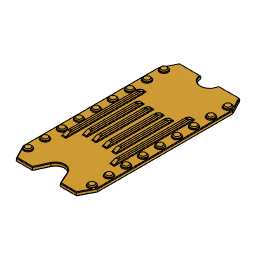
Spojka v7 (Autodesk Fusion 360 design; units mm, degrees)
Autodesk Fusion 360 part; units mm, degrees
note: some values were not read from the file. Set by a fixed rule: which sketch regions a step uses.
sketch "Sketch1" plane through (0, 0, 0) normal (0, 0, 1) x (1, 0, 0)
  line L0 (13.175, -28.845) -> (-13.175, -28.845)
  line L1 (-13.175, -28.845) -> (-13.175, 28.845)
  line L2 (-13.175, 28.845) -> (13.175, 28.845)
  line L3 (13.175, 28.845) -> (13.175, -28.845)
  line L4 (13.175, -28.845) -> (-13.175, 28.845) construction
  line L5 (-13.175, -28.845) -> (13.175, 28.845) construction
  circle A0 centre (0, 28.845) radius 3.15
  circle A1 centre (0, -25.665) radius 3.15
  line L6 (-2.869, -24.3645) -> (-4.9, -28.845)
  line L7 (2.869, -24.3645) -> (4.9, -28.845)
  line L8 (-13.175, 23.845) -> (-10.595, 28.845)
  line L9 (0, 2.5) -> (0, 20)
  line L10 (13.175, 23.845) -> (10.595, 28.845)
  line L11 (20, 0) -> (2.5, 0)
  line L12 (-13.175, -23.845) -> (-10.595, -28.845)
  line L13 (13.175, -23.845) -> (10.595, -28.845)
  circle A2 centre (-11.295, 0) radius 1.25
  circle A3 centre (-11.295, -24) radius 1.25
  circle A4 centre (-11.295, -18) radius 1.25
  circle A5 centre (-11.295, -12) radius 1.25
  circle A6 centre (-11.295, -6) radius 1.25
  circle A7 centre (-11.295, 6) radius 1.25
  circle A8 centre (-11.295, 12) radius 1.25
  circle A9 centre (-11.295, 18) radius 1.25
  circle A10 centre (-11.295, 24) radius 1.25
  circle A11 centre (11.295, 24) radius 1.25
  circle A12 centre (11.295, 18) radius 1.25
  circle A13 centre (11.295, 12) radius 1.25
  circle A14 centre (11.295, 6) radius 1.25
  circle A15 centre (11.295, 0) radius 1.25
  circle A16 centre (11.295, -6) radius 1.25
  circle A17 centre (11.295, -12) radius 1.25
  circle A18 centre (11.295, -18) radius 1.25
  circle A19 centre (11.295, -24) radius 1.25
  line L14 (-7.925, -14) -> (-9.175, -14)
  line L15 (-9.175, -14) -> (-9.175, 14)
  line L16 (-9.175, 14) -> (-7.925, 14)
  line L17 (-7.925, 14) -> (-7.925, -14)
  line L18 (-7.925, -14) -> (-9.175, 14) construction
  line L19 (-9.175, -14) -> (-7.925, 14) construction
  line L20 (-4.575, -10) -> (-5.825, -10)
  line L21 (-5.825, -10) -> (-5.825, 10)
  line L22 (-5.825, 10) -> (-4.575, 10)
  line L23 (-4.575, 10) -> (-4.575, -10)
  line L24 (-4.575, -10) -> (-5.825, 10) construction
  line L25 (-5.825, -10) -> (-4.575, 10) construction
  line L26 (-1.225, -10) -> (-2.475, -10)
  line L27 (-2.475, -10) -> (-2.475, 10)
  line L28 (-2.475, 10) -> (-1.225, 10)
  line L29 (-1.225, 10) -> (-1.225, -10)
  line L30 (-1.225, -10) -> (-2.475, 10) construction
  line L31 (-2.475, -10) -> (-1.225, 10) construction
  line L32 (9.175, -14) -> (9.175, 14)
  line L33 (9.175, 14) -> (7.925, 14)
  line L34 (7.925, -14) -> (9.175, -14)
  line L35 (7.925, 14) -> (7.925, -14)
  line L36 (4.575, 10) -> (4.575, -10)
  line L37 (4.575, -10) -> (5.825, -10)
  line L38 (5.825, 10) -> (4.575, 10)
  line L39 (5.825, -10) -> (5.825, 10)
  line L40 (1.225, 10) -> (1.225, -10)
  line L41 (1.225, -10) -> (2.475, -10)
  line L42 (2.475, 10) -> (1.225, 10)
  line L43 (2.475, -10) -> (2.475, 10)
  point P0 (-8.55, 0)
  point P1 (-5.2, 0)
  point P2 (-1.85, 0)
  dimension "d1" = 26.35
  dimension "d2" = 57.69
  dimension "d3" = 6.3
  dimension "d4" = 9.8
  dimension "d5" = 6.33
  dimension "d6" = 2.58
  dimension "d7" = 5
  dimension "d8" = 2.5
  dimension "d9" = 1.88
  dimension "d12" = 0
  dimension "d13" = 6
  dimension "d14" = 1.25
  dimension "d15" = 28
  dimension "d16" = 1.25
  dimension "d17" = 20
  dimension "d18" = 4
  dimension "d19" = 2.1
  dimension "d20" = 2.1
  constraint horizontal L0
  constraint perpendicular L0 L1
  constraint parallel L0 L2
  constraint parallel L1 L3
  constraint coincident L4 origin
  constraint coincident L5 origin
  constraint midpoint L2 A0.centre
  constraint equal A0 A1
  constraint coincident A1 L6.start
  constraint coincident L0 L6.end
  constraint coincident A1 L7.start
  constraint coincident L0 L7.end
  constraint tangent A1 L7
  constraint tangent A1 L6
  constraint equal L6 L7
  constraint vertical origin A1.centre
  constraint coincident L1 L8.start
  constraint coincident L2 L8.end
  constraint symmetric L8.start L9 L10.start
  constraint symmetric L8.end L9 L10.end
  constraint symmetric L8.start L11 L12.start
  constraint symmetric L8.end L11 L12.end
  constraint symmetric L10.start L11 L13.start
  constraint symmetric L10.end L11 L13.end
  constraint horizontal origin A2.centre
  constraint symmetric L9 A2 A15
  constraint symmetric L9 A3 A19
  constraint symmetric L9 A4 A18
  constraint symmetric L9 A5 A17
  constraint symmetric L9 A6 A16
  constraint symmetric L9 A7 A14
  constraint symmetric L9 A8 A13
  constraint symmetric L9 A9 A12
  constraint symmetric L9 A10 A11
  constraint horizontal L14
  constraint perpendicular L14 L15
  constraint parallel L14 L16
  constraint parallel L15 L17
  constraint coincident L18 P0
  constraint coincident L19 P0
  constraint horizontal L20
  constraint perpendicular L20 L21
  constraint parallel L20 L22
  constraint parallel L21 L23
  constraint coincident L24 P1
  constraint coincident L25 P1
  constraint horizontal origin P1
  constraint horizontal origin P0
  constraint horizontal L26
  constraint perpendicular L26 L27
  constraint parallel L26 L28
  constraint parallel L27 L29
  constraint coincident L30 P2
  constraint coincident L31 P2
  constraint horizontal origin P2
  constraint equal L22 L28
  constraint equal L23 L27
  constraint symmetric L9 L14.start L34.start
  constraint symmetric L9 L14.end L32.start
  constraint symmetric L9 L15.end L32.end
  constraint symmetric L9 L16.end L33.end
  constraint symmetric L9 L20.start L36.end
  constraint symmetric L9 L20.end L37.end
  constraint symmetric L9 L21.end L38.start
  constraint symmetric L9 L22.end L36.start
  constraint symmetric L9 L26.start L40.end
  constraint symmetric L9 L26.end L41.end
  constraint symmetric L9 L27.end L42.start
  constraint symmetric L9 L28.end L40.start
  measures "d1" distance of L1.end L2.end
  measures "d2" distance of L0.end L1.end
  measures "d3" diameter of A0
  measures "d4" distance of L6.end L7.end
  measures "d6" distance of L1.end L8.end
  measures "d7" distance of L1.end L8.start
  measures "d8" diameter of A2
  measures "d9" distance of L1 A2.centre
  measures "d14" distance of L15.end L16.end
  measures "d15" distance of L14.end L15.end
  measures "d16" distance of L21.end L22.end
  measures "d17" distance of L20.end L21.end
  measures "d18" distance of L1 L15
  measures "d19" distance of L17 L21
  measures "d20" distance of L23 L27
extrude "Extrude1" add sketch "Sketch1" along normal blind 1.25 contours L0 L1 L2 L3 A0 A1 L6 L7 L8 L10 L12 L13
extrude "Extrude2" add sketch "Sketch1" along normal blind 1.86 contours L11 A15 | L11 A15 | A2 | A3 | A4 | A5 | A6 | A7 | A8 | A9 | A10 | A11 | A12 | A13 | A14 | A16 | A17 | A18 | A19
extrude "Extrude3" add sketch "Sketch1" along normal blind 2.38 contours L11 L32 L34 L35 | L11 L32 L33 L35 | L11 L36 L37 L39 | L11 L36 L38 L39 | L14 L15 L16 L17 | L20 L21 L22 L23 | L26 L27 L28 L29 | L40 L41 L42 L43
chamfer "Chamfer1" distance 2 distance2 0.9 12 edges at (-8.55, -14, 2.38) (-5.2, -10, 2.38) (-1.85, -10, 2.38) (1.85, -10, 2.38) (5.2, -10, 2.38) (8.55, -14, 2.38) (-5.2, 10, 2.38) (-8.55, 14, 2.38) (-1.85, 10, 2.38) (1.85, 10, 2.38) (5.2, 10, 2.38) (8.55, 14, 2.38) measured on face at (-8.7583, 4.6667, 2.38) measured on face at (-5.4083, 3.3333, 2.38) measured on face at (-2.0583, 3.3333, 2.38) measured on face at (1.6417, 3.3333, 2.38) measured on face at (4.9917, -3.3333, 2.38) measured on face at (8.3417, -4.6667, 2.38) measured on face at (-5.4083, 3.3333, 2.38) measured on face at (-8.7583, 4.6667, 2.38) measured on face at (-2.0583, 3.3333, 2.38) measured on face at (1.6417, 3.3333, 2.38) measured on face at (4.9917, -3.3333, 2.38) measured on face at (8.3417, -4.6667, 2.38)
chamfer "Chamfer2" distance 0.2 distance2 0.2 2 faces at (-3.1285, 16.5679, 1.25) (4.6199, 9.0005, 0)
chamfer "Chamfer2" distance 0.3 distance2 0.3 18 faces at (-10.8968, -24.2388, 1.86) (-10.8968, -18.2388, 1.86) (-10.9095, -12.4155, 1.86) (-11.3501, -5.6896, 1.86) (-11.4611, 0.5728, 1.86) (-11.3501, 6.3104, 1.86) (-10.9095, 11.5845, 1.86) (-10.8968, 17.7612, 1.86) (-10.8968, 23.7612, 1.86) (11.6932, -24.2388, 1.86) (11.6932, -18.2388, 1.86) (11.6805, -12.4155, 1.86) (11.2399, -5.6896, 1.86) (10.9507, 0.2347, 1.86) (11.2399, 6.3104, 1.86) (11.6805, 11.5845, 1.86) (11.6932, 17.7612, 1.86) (11.6932, 23.7612, 1.86)
chamfer "Chamfer2" distance 0.3 distance2 0.3 6 faces at (-8.7583, 4, 2.38) (-5.4083, 2.6667, 2.38) (-2.0583, 2.6667, 2.38) (1.6417, 2.6667, 2.38) (4.9917, -2.6667, 2.38) (8.7583, 4, 2.38)
equation "d20 = d19"
named bodies: "Spojka"
